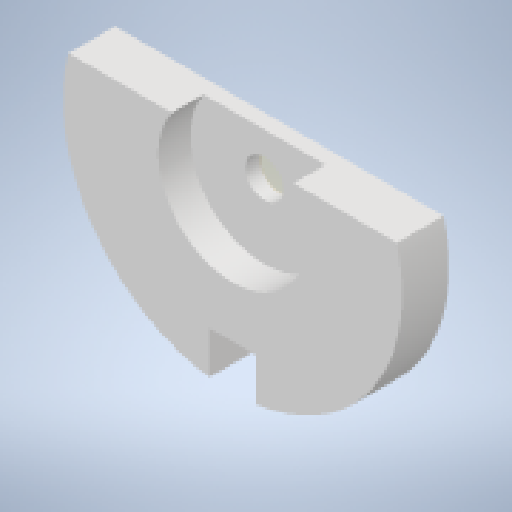
# Autodesk Inventor part: circle
Saved by Autodesk Inventor 2023 (Build 270158000, 158)
## iProperties
Created: 2026-02-13
Part Number: circle
Material: Типовые
Document SubType Name: Modeling
Designer: garin
Density: 1 g/cm^3
Appearance: По умолчанию
Author: garin
Autodesk Inventor part; units mm, degrees
ref_plane "YZ Plane" through (0, 0, 0) normal (1, 0, 0) x (0, 1, 0)
ref_plane "XZ Plane" through (0, 0, 0) normal (0, 1, 0) x (-1, 0, 0)
ref_plane "XY Plane" through (0, 0, 0) normal (0, 0, 1) x (1, 0, 0)
sketch "Эскиз1" plane through (0, 0, 0) normal (0, 0, 1) x (1, 0, 0)
  line L0 (0, 0) -> (-6, 0) construction
  line L1 (-6, 0) -> (-6, -27.9727) construction
  line L2 (-6, -27.9727) -> (0, -27.9727) construction
  line L3 (0, -27.9727) -> (0, 0) construction
  line L4 (6, -39.5474) -> (6, -29.5474)
  line L5 (6, -29.5474) -> (-6, -29.5474)
  line L6 (-6, -29.5474) -> (-6, -39.5474)
  circle A0 centre (0, 0) radius 4.45
  circle A1 centre (0, 0) radius 40
  line L7 (29.5474, -6) -> (39.5474, -6)
  line L8 (29.5474, 6) -> (29.5474, -6)
  line L9 (39.5474, 6) -> (29.5474, 6)
  line L10 (6, 29.5474) -> (6, 39.5474)
  line L11 (-6, 29.5474) -> (6, 29.5474)
  line L12 (-6, 39.5474) -> (-6, 29.5474)
  line L13 (-29.5474, 6) -> (-39.5474, 6)
  line L14 (-29.5474, -6) -> (-29.5474, 6)
  line L15 (-39.5474, -6) -> (-29.5474, -6)
  line L16 (38.7298, 10) -> (-38.7298, 10)
  circle A2 centre (0, 0) radius 17.5
  line L17 (0, -40) -> (0, -29.6)
  line L18 (0, -29.6) -> (-6, -29.6)
  line L19 (0, -29.6) -> (6, -29.6)
  line L20 (5.5, -29.5474) -> (5.5, -39.6201)
  line L21 (-5.5, -29.5474) -> (-5.5, -39.6201)
  point P0 (6, -34.4819)
  point P1 (6, -27.9727)
  point P2 (6, -39.5474)
  point P3 (6, -39.5474)
  point P4 (-14.3614, 10)
  point P5 (14.3614, 10)
  point P6 (5.5, -29.6)
  point P7 (-5.5, -29.6)
  dimension "d1" = 6
  dimension "d2" = 12
  dimension "d3" = 10
  dimension "d6" = 8.9
  dimension "d12" = 80
  dimension "d15" = 360
  dimension "d19" = 35
  dimension "d24" = 10.4
  dimension "d25" = 0.5
  constraints: 44 end point, 5 point on circle, 3 centre point, 3 coincident, 3 parallel, 3 perpendicular, 3 point on line, 2 horizontal, 2 symmetric about line, 1 vertical, 29 other
  measures "d1" distance of L2.start L2.end
  measures "d2" distance of L5.end L4.end
  measures "d3" distance of L4.end L4.start
  measures "d6" diameter of A0
  measures "d12" diameter of A1
  measures "d19" diameter of A2
  measures "d24" distance of L17.start L17.end
  measures "d25" distance of L4.end L20.start
ref_plane "РабПлоскость2" through (0, 0, 0.2) normal (0, 0, 1) x (1, 0, 0)
extrude "Выдавливание4" add sketch "Эскиз1" along normal blind 3.5 contours A2 L16 picked at (-0.1788, 8.1392)
extrude "Выдавливание5" add sketch "Эскиз1" along normal blind 11 contours A1 L20 L19 L4 | L4 L5 L6 A1 L15 L14 L13 L16 A2 L9 L8 L7 | L19 L20 L5 L4 | L7 L8 L9 A1 | A1 L6 L18 L21 | L21 L18 L6 L5 | A1 L13 L14 L15
fillet "Сопряжение1" radius 1 2 edges at (14.3614, 10, 7.25) (-14.3614, 10, 7.25)
